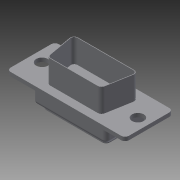
# Autodesk Inventor part: DSUB_9_Male
Saved by Autodesk Inventor 2014 (Build 180170000, 170)
## iProperties
Created: 2015-11-07
Part Number: DSUB_9_Male
Material: Generic
Document SubType Name: Modeling
Designer: Owner
Density: 1 g/cm^3
Appearance: Default
Author: Owner
Autodesk Inventor part; units mm, degrees
ref_plane "YZ Plane" through (0, 0, 0) normal (1, 0, 0) x (0, 1, 0)
ref_plane "XZ Plane" through (0, 0, 0) normal (0, 1, 0) x (-1, 0, 0)
ref_plane "XY Plane" through (0, 0, 0) normal (0, 0, 1) x (1, 0, 0)
sketch "Sketch1" plane through (0, 0, 0) normal (0, 1, 0) x (-1, 0, 0)
  line L0 (-14.405, 6.275) -> (14.405, 6.275)
  line L1 (15.405, 5.275) -> (15.405, -5.275)
  line L2 (14.405, -6.275) -> (-14.405, -6.275)
  line L3 (-15.405, -5.275) -> (-15.405, 5.275)
  arc A0 (-14.405, 6.275) -> (-15.405, 5.275) centre (-14.405, 5.275) ccw
  arc A1 (15.405, 5.275) -> (14.405, 6.275) centre (14.405, 5.275) ccw
  arc A2 (14.405, -6.275) -> (15.405, -5.275) centre (14.405, -5.275) ccw
  arc A3 (-15.405, -5.275) -> (-14.405, -6.275) centre (-14.405, -5.275) ccw
  circle A4 centre (12.495, 0) radius 1.525
  circle A5 centre (-12.495, 0) radius 1.525
  point P0 (0, 0)
  point P1 (-15.405, 6.275)
  point P2 (15.405, -6.275)
  point P3 (15.405, 6.275)
  dimension "d0" = 30.81
  dimension "d1" = 12.55
  dimension "d2" = 6.275
  dimension "d3" = 15.405
  dimension "d4" = 1
  dimension "d16" = 3.05
  dimension "d17" = 3.05
  dimension "d18" = 24.99
  dimension "d19" = 12.495
  constraints: 8 end point, 8 point on circle, 8 tangent, 6 centre point, 6 point on line, 3 equal radius, 2 parallel, 1 horizontal, 1 perpendicular
  measures "d0" distance of point (-15.405, 6.275) point (15.405, 6.275)
  measures "d1" distance of point (15.405, 6.275) point (15.405, -6.275)
  measures "d2" distance from line of point (0, 0) L0
  measures "d3" distance from line of L1 point (0, 0)
  measures "d4" radius of A0
  measures "d16" diameter of A5
  measures "d17" diameter of A4
  measures "d18" distance of A5.centre A4.centre
  measures "d19" distance of A5.centre point (0, 0)
extrude "Extrusion1" add sketch "Sketch1" along normal blind 1
sketch "Sketch2" plane through (0, 1, 0) normal (0, 1, 0) x (1, 0, 0)
  line L0 (-7.3082, 4.18) -> (7.3082, 4.18)
  line L1 (8.5, 4.18) -> (8.5, -4.18)
  line L2 (6.1868, -4.18) -> (-6.1868, -4.18)
  line L3 (-8.5, -4.18) -> (-8.5, 4.18)
  line L4 (-8.2931, 3.0064) -> (-7.1716, -3.3536)
  line L5 (8.2931, 3.0064) -> (7.1716, -3.3536)
  arc A0 (-7.3082, 4.18) -> (-8.2931, 3.0064) centre (-7.3082, 3.18) ccw
  arc A1 (-7.1716, -3.3536) -> (-6.1868, -4.18) centre (-6.1868, -3.18) ccw
  arc A2 (6.1868, -4.18) -> (7.1716, -3.3536) centre (6.1868, -3.18) ccw
  arc A3 (8.2931, 3.0064) -> (7.3082, 4.18) centre (7.3082, 3.18) ccw
  line L6 (7.3082, 4.0255) -> (-7.3082, 4.0255)
  arc A4 (-7.3082, 4.0255) -> (-8.1409, 3.0332) centre (-7.3082, 3.18) ccw
  line L7 (-8.1409, 3.0332) -> (-7.0195, -3.3268)
  arc A5 (-7.0195, -3.3268) -> (-6.1868, -4.0255) centre (-6.1868, -3.18) ccw
  line L8 (-6.1868, -4.0255) -> (6.1868, -4.0255)
  arc A6 (6.1868, -4.0255) -> (7.0195, -3.3268) centre (6.1868, -3.18) ccw
  line L9 (7.0195, -3.3268) -> (8.1409, 3.0332)
  arc A7 (8.1409, 3.0332) -> (7.3082, 4.0255) centre (7.3082, 3.18) ccw
  point P0 (0, 0)
  dimension "d7" = 17
  dimension "d8" = 8.36
  dimension "d9" = 4.18
  dimension "d10" = 8.5
  dimension "d11" = 10
  dimension "d12" = 10
  dimension "d13" = 1
  constraints: 20 end point, 16 point on circle, 8 centre point, 8 tangent, 6 point on line, 3 equal radius, 3 parallel, 1 horizontal, 1 perpendicular, 7 other
  measures "d7" distance of L3.end L1.start
  measures "d8" distance of L1.start L1.end
  measures "d9" distance from line of point (0, 0) L0
  measures "d10" distance from line of L1 point (0, 0)
  measures "d11" angle of L1 L5
  measures "d12" angle of L3 L4
  measures "d13" radius of A0
extrude "Extrusion2" add sketch "Sketch2" along normal blind 6.1
sketch "Sketch3" plane through (0, 0, 0) normal (0, -1, 0) x (1, 0, 0)
  line L0 (-8.6, 5.36) -> (8.6, 5.36)
  line L1 (9.6, 4.36) -> (9.6, -4.36)
  line L2 (8.6, -5.36) -> (-8.6, -5.36)
  line L3 (-9.6, -4.36) -> (-9.6, 4.36)
  arc A0 (-8.6, 5.36) -> (-9.6, 4.36) centre (-8.6, 4.36) ccw
  arc A1 (9.6, 4.36) -> (8.6, 5.36) centre (8.6, 4.36) ccw
  arc A2 (8.6, -5.36) -> (9.6, -4.36) centre (8.6, -4.36) ccw
  arc A3 (-9.6, -4.36) -> (-8.6, -5.36) centre (-8.6, -4.36) ccw
  point P0 (0, 0)
  point P1 (-9.6, 5.36)
  point P2 (9.6, -5.36)
  point P3 (9.6, 5.36)
  dimension "d20" = 19.2
  dimension "d21" = 10.72
  dimension "d22" = 5.36
  dimension "d23" = 9.6
  dimension "d24" = 1
  constraints: 8 end point, 8 point on circle, 8 tangent, 6 point on line, 4 centre point, 3 equal radius, 2 parallel, 1 horizontal, 1 perpendicular
  measures "d20" distance of point (-9.6, 5.36) point (9.6, 5.36)
  measures "d21" distance of point (9.6, 5.36) point (9.6, -5.36)
  measures "d22" distance from line of point (0, 0) L0
  measures "d23" distance from line of L3 point (0, 0)
  measures "d24" radius of A0
extrude "Extrusion3" add sketch "Sketch3" along normal blind 4.1
fillet "Fillet1" radius 0.9 8 edges at (9.3071, -4.1, -5.0671) (9.6, -4.1, 0) (9.3071, -4.1, 5.0671) (0, -4.1, 5.36) (-9.3071, -4.1, 5.0671) (-9.6, -4.1, 0) (-9.3071, -4.1, -5.0671) (0, -4.1, -5.36)
sketch "Sketch4" plane through (0, -4.1, 0) normal (0, -1, 0) x (1, 0, 0)
  line L0 (-7.2476, 4.1431) -> (7.3248, 4.1431)
  line L1 (8.3248, 3.1431) -> (8.3248, -3.1174)
  line L2 (7.3248, -4.1174) -> (-7.2476, -4.1174)
  line L3 (-8.2476, -3.1174) -> (-8.2476, 3.1431)
  arc A0 (-7.2476, 4.1431) -> (-8.2476, 3.1431) centre (-7.2476, 3.1431) ccw
  arc A1 (8.3248, 3.1431) -> (7.3248, 4.1431) centre (7.3248, 3.1431) ccw
  arc A2 (7.3248, -4.1174) -> (8.3248, -3.1174) centre (7.3248, -3.1174) ccw
  arc A3 (-8.2476, -3.1174) -> (-7.2476, -4.1174) centre (-7.2476, -3.1174) ccw
  point P0 (0, 0)
  point P1 (-8.2476, 4.1431)
  point P2 (8.3248, -4.1174)
  point P3 (8.3248, 4.1431)
  point P4 (-8.2476, -4.1174)
  dimension "d30" = 1
  constraints: 8 end point, 8 point on circle, 8 point on line, 8 tangent, 4 centre point, 3 equal radius, 2 parallel, 1 horizontal, 1 perpendicular
  measures "d30" radius of A0
extrude "Extrusion4" add sketch "Sketch4" along normal blind 1
body "Solid1"
